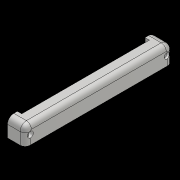
# Autodesk Inventor part: small_gpu_03
Saved by Autodesk Inventor 2018.2 (Build 222227000, 227)
## iProperties
Created: 2020-06-13
Part Number: small_gpu_03
Material: アルミニウム 6061
Document SubType Name: Modeling
Designer: gisen
Density: 2.7 g/cm^3
Appearance: アルミニウム - フラット
Author: gisen
Autodesk Inventor part; units mm, degrees
ref_plane "YZ Plane" through (0, 0, 0) normal (1, 0, 0) x (0, 1, 0)
ref_plane "XZ Plane" through (0, 0, 0) normal (0, 1, 0) x (-1, 0, 0)
ref_plane "XY Plane" through (0, 0, 0) normal (0, 0, 1) x (1, 0, 0)
sketch "スケッチ1" plane through (0, 0, 0) normal (0, 0, 1) x (1, 0, 0)
  line L0 (0, 0) -> (14, 0)
  line L1 (14, 0) -> (14, 117)
  line L2 (14, 117) -> (0, 117)
  line L3 (0, 117) -> (0, 109.16)
  line L4 (0, 109.16) -> (3.5, 109.16)
  line L5 (3.5, 109.16) -> (3.5, 7.84)
  line L6 (3.5, 7.84) -> (0, 7.84)
  line L7 (0, 7.84) -> (0, 0)
  dimension "d0" = 117
  dimension "d1" = 3.5
  dimension "d2" = 7.84
  dimension "d3" = 14
  constraints: 16 end point, 6 perpendicular, 1 collinear, 1 horizontal, 1 point on line, 1 vertical
  measures "d0" distance of L0.end L1.end
  measures "d1" distance between parallel lines of L7 L5
  measures "d2" distance of L2.end L3.end
  measures "d3" distance of L1.end L2.end
extrude "押し出し1" add sketch "スケッチ1" along normal blind 14.4
sketch "スケッチ2" plane through (0, 0, 0) normal (-1, 0, 0) x (0, 0, 1)
  line L0 (0, 117) -> (14.4, 117) construction
  line L1 (0, 0) -> (14.4, 0) construction
  line L2 (0, 117) -> (14.4, 117) construction
  line L3 (7.15, 117) -> (7.15, 0) construction
  line L4 (0, 0) -> (14.4, 0) construction
  circle A0 centre (7.15, 4.35) radius 1.8 construction
  line L5 (7.15, 4.35) -> (5.35, 4.35) construction
  line L6 (0, 7.84) -> (0, 0) construction
  circle A1 centre (7.15, 4.35) radius 2.25
  line L7 (7.15, 58.5) -> (14.4, 58.5) construction
  line L8 (14.4, 0) -> (14.4, 117) projected
  circle A2 centre (7.15, 112.65) radius 2.25
  point P0 (7.15, 2.55)
  dimension "d6" = 3.6
  dimension "d7" = 5.35
  dimension "d8" = 2.55
  dimension "d9" = 4.5
  constraints: 6 end point, 4 point on line, 3 centre point, 2 midpoint, 2 point on circle, 1 coincident, 1 horizontal, 1 perpendicular, 1 symmetric about line, 1 other
  measures "d6" diameter of A0
  measures "d7" distance from line of L6 L5.end
  measures "d8" distance from line of L1 A0.end
  measures "d9" diameter of A1
extrude "押し出し2" cut sketch "スケッチ2" against normal through all
fillet "フィレット1" radius 5 2 edges at (7, 0, 14.4) (7, 117, 14.4)
sketch "スケッチ3" plane through (0, 0, 0) normal (0, 0, -1) x (-1, 0, 0)
  line L0 (0, 7.84) -> (0, 0) construction
  line L1 (-14, 0) -> (-14, 117) construction
  line L2 (0, 117) -> (0, 109.16) construction
  line L3 (0, 3.92) -> (-14, 3.92) construction
  circle A0 centre (-10, 3.92) radius 2.25
  line L4 (-14, 5) -> (-14, 112) construction
  line L5 (-14, 58.5) -> (-3.7036, 58.5) construction
  circle A1 centre (-10, 113.08) radius 2.25
  dimension "d13" = 7.84
  dimension "d14" = 4.5
  dimension "d17" = 4
  constraints: 4 end point, 2 centre point, 2 midpoint, 2 point on line, 1 horizontal, 1 perpendicular, 1 symmetric about line, 1 other
  measures "d13" distance of L0.start L0.end
  measures "d14" diameter of A0
  measures "d17" distance from line of L1 A0.centre
extrude "押し出し3" cut sketch "スケッチ3" against normal blind 7.5
fillet "フィレット2" radius 4 5 edges at (14, 1.4645, 12.9355) (14, 58.5, 14.4) (14, 115.5355, 12.9355) (14, 117, 4.7) (14, 0, 4.7)
